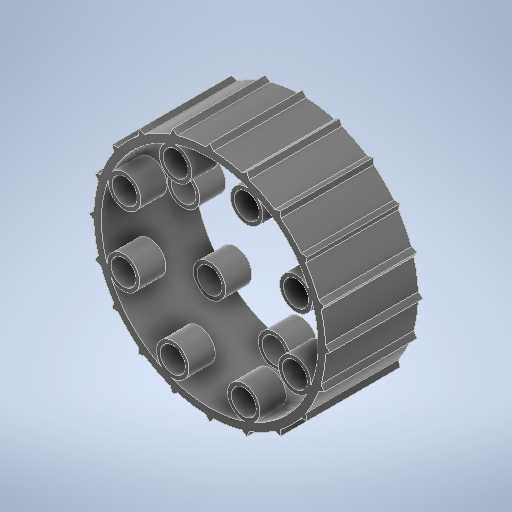
# Autodesk Inventor part: opona
Saved by Autodesk Inventor 2025.3 (Build 293356000, 356)
## iProperties
Created: 2026-03-13
Part Number: opona
Material: Thermoplastic Resin
Document SubType Name: Modeling
Designer: ksawe
Density: 1.28 g/cm^3
Appearance: Smooth - Black
Author: ksawe
Autodesk Inventor part; units mm, degrees
ref_plane "YZ Plane" through (0, 0, 0) normal (1, 0, 0) x (0, 1, 0)
ref_plane "XZ Plane" through (0, 0, 0) normal (0, 1, 0) x (-1, 0, 0)
ref_plane "XY Plane" through (0, 0, 0) normal (0, 0, 1) x (1, 0, 0)
sketch "Sketch1" plane through (0, 0, 0) normal (0, 0, 1) x (1, 0, 0)
  circle A0 centre (0, 0) radius 75
  circle A1 centre (0, 0) radius 70
  dimension "d0" = 150
  dimension "d1" = 140
  constraints: 2 centre point, 2 coincident
  measures "d0" diameter of A0
  measures "d1" diameter of A1
extrude "Extrusion1" add sketch "Sketch1" along normal mid plane 60
sketch "Sketch2" plane through (0, 0, 30) normal (0, 0, 1) x (1, 0, 0)
  circle A0 centre (0, 0) radius 50
  circle A1 centre (0, 0) radius 70 projected
  circle A2 centre (1, 60) radius 10.5
  circle A3 centre (1, 60) radius 8
  circle A4 centre (-22.0371, 55.8155) radius 8
  circle A5 centre (-22.0371, 55.8155) radius 10.5
  circle A6 centre (-41.7193, 43.1335) radius 8
  circle A7 centre (-41.7193, 43.1335) radius 10.5
  circle A8 centre (-55.0501, 23.8849) radius 8
  circle A9 centre (-55.0501, 23.8849) radius 10.5
  circle A10 centre (-60, 1) radius 8
  circle A11 centre (-60, 1) radius 10.5
  circle A12 centre (-55.8155, -22.0371) radius 8
  circle A13 centre (-55.8155, -22.0371) radius 10.5
  circle A14 centre (-43.1335, -41.7193) radius 8
  circle A15 centre (-43.1335, -41.7193) radius 10.5
  circle A16 centre (-23.8849, -55.0501) radius 8
  circle A17 centre (-23.8849, -55.0501) radius 10.5
  circle A18 centre (-1, -60) radius 8
  circle A19 centre (-1, -60) radius 10.5
  circle A20 centre (22.0371, -55.8155) radius 8
  circle A21 centre (22.0371, -55.8155) radius 10.5
  circle A22 centre (41.7193, -43.1335) radius 8
  circle A23 centre (41.7193, -43.1335) radius 10.5
  circle A24 centre (55.0501, -23.8849) radius 8
  circle A25 centre (55.0501, -23.8849) radius 10.5
  circle A26 centre (60, -1) radius 8
  circle A27 centre (60, -1) radius 10.5
  circle A28 centre (55.8155, 22.0371) radius 8
  circle A29 centre (55.8155, 22.0371) radius 10.5
  circle A30 centre (43.1335, 41.7193) radius 8
  circle A31 centre (43.1335, 41.7193) radius 10.5
  circle A32 centre (23.8849, 55.0501) radius 8
  circle A33 centre (23.8849, 55.0501) radius 10.5
  point P0 (-2.3192, 69.9616)
  point P1 (4.6493, 69.8454)
  point P2 (-28.9158, 63.7485)
  point P3 (-22.4333, 66.308)
  point P4 (-46.1006, 52.6757)
  point P5 (-51.1102, 47.8304)
  point P6 (-62.7495, 31.0241)
  point P7 (-65.5236, 24.6305)
  point P8 (-69.8454, 4.6493)
  point P9 (-69.9616, -2.3192)
  point P10 (-66.308, -22.4333)
  point P11 (-63.7485, -28.9158)
  point P12 (-24.6305, -65.5236)
  point P13 (-31.0241, -62.7495)
  point P14 (-47.8304, -51.1102)
  point P15 (-52.6757, -46.1006)
  point P16 (22.4333, -66.308)
  point P17 (28.9158, -63.7485)
  point P18 (62.7495, -31.0241)
  point P19 (65.5236, -24.6305)
  point P20 (63.7485, 28.9158)
  point P21 (66.308, 22.4333)
  point P22 (24.6305, 65.5236)
  point P23 (31.0241, 62.7495)
  dimension "d4" = 100
  dimension "d10" = 2.5
  dimension "d13" = 360
  dimension "d52" = 60
  dimension "d53" = 22.8849
  dimension "d105" = 16
  constraints: 33 centre point, 3 coincident, 50 other
  measures "d4" diameter of A0
  measures "d10" radial gap between concentric circles of A2 A3
  measures "d52" vertical distance of point (0, 0) A2.centre
  measures "d53" horizontal distance of A32.centre A2.centre
  measures "d105" diameter of A3
extrude "Extrusion3" add sketch "Sketch2" against normal blind 17 contours A29 A0 | A0 A29 A1 | A25 A1 A0 | A0 A25 | A33 A0 | A0 A33 A1 | A21 A1 A0 | A0 A21 | A5 A0 | A0 A5 A1 | A17 A1 A0 | A0 A17 | A9 A0 | A0 A9 A1 | A13 A1 A0 | A0 A13
sketch "Sketch4" plane through (0, 0, -30) normal (0, 0, -1) x (-1, 0, 0)
  circle A0 centre (22.0371, 55.8155) radius 8 projected
  arc A1 (22.4333, 66.308) -> (28.9158, 63.7485) centre (22.0371, 55.8155) ccw projected
  circle A2 centre (22.0371, 55.8155) radius 8
  circle A3 centre (22.0371, 55.8155) radius 10.5
  circle A4 centre (-0.9999, 60.0006) radius 10.5
  circle A5 centre (-0.9999, 60.0006) radius 8
  circle A6 centre (-23.8849, 55.0512) radius 10.5
  circle A7 centre (-23.8849, 55.0512) radius 8
  circle A8 centre (-43.1338, 41.7209) radius 10.5
  circle A9 centre (-43.1338, 41.7209) radius 8
  circle A10 centre (-55.8163, 22.0391) radius 10.5
  circle A11 centre (-55.8163, 22.0391) radius 8
  circle A12 centre (-60.0014, -0.9979) radius 10.5
  circle A13 centre (-60.0014, -0.9979) radius 8
  circle A14 centre (-55.0521, -23.8829) radius 10.5
  circle A15 centre (-55.0521, -23.8829) radius 8
  circle A16 centre (-41.7218, -43.1319) radius 10.5
  circle A17 centre (-41.7218, -43.1319) radius 8
  circle A18 centre (-22.0399, -55.8143) radius 10.5
  circle A19 centre (-22.0399, -55.8143) radius 8
  circle A20 centre (0.9971, -59.9994) radius 10.5
  circle A21 centre (0.9971, -59.9994) radius 8
  circle A22 centre (23.8821, -55.0501) radius 10.5
  circle A23 centre (23.8821, -55.0501) radius 8
  circle A24 centre (43.1311, -41.7198) radius 10.5
  circle A25 centre (43.1311, -41.7198) radius 8
  circle A26 centre (55.8135, -22.0379) radius 10.5
  circle A27 centre (55.8135, -22.0379) radius 8
  circle A28 centre (59.9986, 0.9991) radius 10.5
  circle A29 centre (59.9986, 0.9991) radius 8
  circle A30 centre (55.0493, 23.8841) radius 10.5
  circle A31 centre (55.0493, 23.8841) radius 8
  circle A32 centre (41.719, 43.133) radius 10.5
  circle A33 centre (41.719, 43.133) radius 8
  point P0 (-0.0014, 0.0006)
  dimension "d108" = 360
  dimension "d110" = 2.5
  dimension "d111" = 16
  dimension "d112" = 22.885
  dimension "d113" = 60
  constraints: 32 centre point, 17 coincident, 65 other
  measures "d110" radial gap between concentric circles of A5 A4
  measures "d111" diameter of A5
  measures "d112" horizontal distance of A6.centre A4.centre
  measures "d113" vertical distance of A4.centre point (-0.001, 0.001)
extrude "Extrusion4" add sketch "Sketch4" against normal blind 17 contours A4 | A8 | A12 | A16 | A20 | A24 | A28 | A32
sketch "Sketch5" plane through (0, 0, 30) normal (0, 0, 1) x (1, 0, 0)
  circle A0 centre (0, 0) radius 75 projected
  circle A1 centre (0, 0) radius 75 projected
  line L0 (2.5, 74.9583) -> (0, 78)
  line L1 (0, 78) -> (-2.5, 74.9583)
  point P0 (-2.5, 74.9583)
  point P1 (2.5, 74.9583)
  dimension "d115" = 78
  dimension "d116" = 5
  constraints: 4 end point, 2 point on circle, 1 equal length, 1 vertical alignment
  measures "d115" distance of A0.centre L0.end
  measures "d116" distance of L0.start L1.end
extrude "Extrusion5" add sketch "Sketch5" against normal blind 60 contours A0 L1 L0
pattern_circular "Circular Pattern1" count 20 over 360 about axis through (0, 0, 0) along (0, 0, 1) of "Extrusion5"
body "Solid1"
